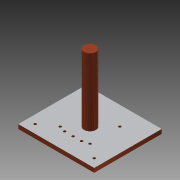
# Autodesk Inventor part: 知能ロボコンばね受け受け
Saved by Autodesk Inventor 2013 (Build 170138000, 138)
## iProperties
Created: 2014-05-15
Part Number: 知能ロボコンばね受け受け
Material: ABS プラスチック
Document SubType Name: Modeling
Designer: horumo136
Density: 1 g/cm^3
Author: horumo136
Autodesk Inventor part; units mm, degrees
ref_plane "YZ Plane" through (0, 0, 0) normal (1, 0, 0) x (0, 1, 0)
ref_plane "XZ Plane" through (0, 0, 0) normal (0, 1, 0) x (-1, 0, 0)
ref_plane "XY Plane" through (0, 0, 0) normal (0, 0, 1) x (1, 0, 0)
sketch "スケッチ1" plane through (0, 0, 0) normal (0, 0, 1) x (1, 0, 0)
  circle A0 centre (-17.6777, 17.6777) radius 1.5
  circle A1 centre (17.6777, -17.6777) radius 1.5
  circle A2 centre (-17.6777, -17.6777) radius 1.5
  circle A3 centre (17.6777, 17.6777) radius 1.5
  line L0 (45, 40) -> (-45, 40)
  line L1 (-45, 40) -> (-45, -40)
  line L2 (-45, -40) -> (45, -40)
  line L3 (45, -40) -> (45, 40)
  line L4 (-5.5, 19.2289) -> (-5.5, 28)
  line L5 (-5.5, 28) -> (5.5, 28)
  line L6 (5.5, 28) -> (5.5, 19.2289)
  arc A4 (-5.5, 19.2289) -> (5.5, 19.2289) centre (0, 0) ccw
  constraints: 14 end point, 5 centre point, 2 point on circle
extrude "押し出し1" add sketch "スケッチ1" along normal blind 5
sketch "スケッチ2" plane through (0, 0, 0) normal (0, 0, -1) x (-1, 0, 0)
  line L0 (-5.5, 28) -> (5.5, 28) projected
  line L1 (5.5, 28) -> (5.5, 19.2289) projected
  arc A0 (-5.5, 19.2289) -> (5.5, 19.2289) centre (0, 0) ccw projected
  line L2 (-5.5, 19.2289) -> (-5.5, 28) projected
  circle A1 centre (0, 0) radius 20
  line L3 (-5.5, 19.2289) -> (-5.5, 28)
  line L4 (5.5, 28) -> (5.5, 19.2289)
  constraints: 4 end point, 2 collinear, 1 centre point, 1 coincident, 1 concentric
extrude "押し出し2" add sketch "スケッチ2" against normal blind 5 contours L0 L1 A1 L2
sketch "スケッチ3" plane through (0, 0, 0) normal (0, 0, -1) x (-1, 0, 0)
  circle A0 centre (0, 0) radius 20 projected
  circle A1 centre (0, 0) radius 20
  constraints: 1 centre point, 1 coincident, 1 concentric
extrude "押し出し3" add sketch "スケッチ3" against normal blind 5
sketch "スケッチ4" plane through (0, 0, 5) normal (0, 0, 1) x (1, 0, 0)
  line L0 (-45, -40) -> (45, -40) projected
  line L1 (45, -40) -> (45, 40) projected
  line L2 (0, -40) -> (0, -20)
  line L3 (0, -20) -> (-10, -20)
  line L4 (-10, -20) -> (10, -20)
  line L5 (-45, -40) -> (-35, -40)
  line L6 (-35, -40) -> (-35, -30)
  line L7 (-35, -30) -> (-45, -30)
  line L8 (-45, -30) -> (-45, -40)
  line L9 (45, -40) -> (35, -40)
  line L10 (35, -40) -> (35, -30)
  line L11 (35, -30) -> (45, -30)
  line L12 (45, -30) -> (45, -40)
  point P0 (0, 0)
  dimension "d6" = 20
  dimension "d7" = 10
  dimension "d8" = 20
  dimension "d9" = 10
  dimension "d10" = 10
  dimension "d11" = 10
  dimension "d12" = 10
  constraints: 22 end point, 5 coincident, 5 parallel, 3 perpendicular, 2 horizontal, 1 collinear, 1 midpoint
  measures "d6" distance of L2.start L2.end
  measures "d7" distance of L2.end L3.end
  measures "d8" distance of L3.end L4.end
  measures "d9" distance of L7.end L6.end
  measures "d10" distance of L6.end L5.end
  measures "d11" distance of L10.end L11.end
  measures "d12" distance of L9.end L10.end
hole "穴1" at (-35, -30, 5) at (-10, -20, 5) at (0, -20, 5) at (10, -20, 5) at (35, -30, 5) direction (0, 0, -1) diameter 3 depth 8 tip angle 118
sketch "スケッチ5" plane through (0, 0, 5) normal (0, 0, 1) x (1, 0, 0)
  circle A0 centre (0, 0) radius 7
  dimension "d20" = 14
  constraints: 2 coincident, 1 centre point
  measures "d20" diameter of A0
sketch "スケッチ6" plane through (0, 0, 5) normal (0, 0, 1) x (1, 0, 0)
  circle A0 centre (10, -20) radius 1.5 projected
  circle A1 centre (-10, -20) radius 1.5 projected
  circle A2 centre (-35, -30) radius 1.5 projected
  circle A3 centre (0, -20) radius 1.5 projected
  circle A4 centre (35, -30) radius 1.5 projected
  circle A5 centre (17.6777, 17.6777) radius 1.5 projected
  circle A6 centre (-17.6777, -17.6777) radius 1.5 projected
  circle A7 centre (17.6777, -17.6777) radius 1.5 projected
  circle A8 centre (-17.6777, 17.6777) radius 1.5 projected
  line L0 (45, 40) -> (-45, 40) projected
  line L1 (-45, 40) -> (-45, -40) projected
  line L2 (-45, -40) -> (45, -40) projected
  line L3 (45, -40) -> (45, 40) projected
  point P0 (0, 0)
extrude "押し出し4" add sketch "スケッチ5" along normal blind 80
